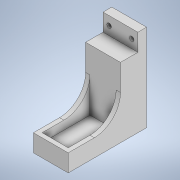
# Autodesk Inventor part: s_base8
Saved by Autodesk Inventor 2022 (Build 260153000, 153)
## iProperties
Created: 2021-09-17
Part Number: s_base8
Material: Generic
Document SubType Name: Modeling
Designer: yuto6
Density: 1 g/cm^3
Appearance: Default
Author: yuto6
Autodesk Inventor part; units mm, degrees
ref_plane "YZ Plane" through (0, 0, 0) normal (1, 0, 0) x (0, 1, 0)
ref_plane "XZ Plane" through (0, 0, 0) normal (0, 1, 0) x (-1, 0, 0)
ref_plane "XY Plane" through (0, 0, 0) normal (0, 0, 1) x (1, 0, 0)
sketch "スケッチ1" plane through (0, 0, 0) normal (1, 0, 0) x (0, 1, 0)
  line L0 (0, 0) -> (100, 0)
  line L1 (100, 0) -> (100, 10)
  line L2 (20, 90) -> (0, 90)
  line L3 (0, 90) -> (0, 0)
  line L4 (100, 10) -> (80, 10)
  line L5 (80, 10) -> (80, 30)
  line L6 (80, 30) -> (20, 30)
  line L7 (20, 30) -> (20, 90)
  dimension "d0" = 100
  dimension "d1" = 10
  dimension "d23" = 20
  dimension "d24" = 20
  dimension "d25" = 80
  dimension "d26" = 90
  constraints: 16 end point, 4 horizontal, 2 perpendicular, 2 vertical
  measures "d0" distance of L0.start L0.end
  measures "d1" distance of L0.end L1.end
  measures "d23" distance of L1.end L4.end
  measures "d24" distance of L4.end L5.end
  measures "d25" distance between parallel lines of L1 L7
  measures "d26" distance between parallel lines of L0 L2
extrude "押し出し1" add sketch "スケッチ1" along normal mid plane 40
fillet "フィレット1" radius 30 1 edges at (0, 20, 30)
sketch "スケッチ2" plane through (-20, 100, 10) normal (0, 1, 0) x (1, 0, 0)
  line L0 (0, -80) -> (40, -80) projected
  line L1 (40, -20) -> (0, -20) projected
  line L2 (5, -20) -> (35, -20)
  line L3 (35, -20) -> (35, -75)
  line L4 (35, -75) -> (5, -75)
  line L5 (5, -75) -> (5, -20)
  line L6 (0, -20) -> (0, -50) projected
  line L7 (40, -50) -> (40, -80) projected
  dimension "d27" = 5
  dimension "d28" = 5
  dimension "d29" = 5
  constraints: 8 end point, 2 parallel, 1 horizontal, 1 perpendicular, 1 point on line
  measures "d27" distance between parallel lines of L0 L4
  measures "d28" distance between parallel lines of L6 L5
  measures "d29" distance between parallel lines of L7 L3
extrude "押し出し2" cut sketch "スケッチ2" against normal blind 90
sketch "スケッチ3" plane through (20, 100, 0) normal (0, 0, -1) x (-1, 0, 0)
  line L0 (40, 0) -> (0, 0) projected
  line L1 (0, -100) -> (0, 0) projected
  line L2 (40, 0) -> (40, -100) projected
  point P0 (20, -100)
  point P1 (7, -10)
  point P2 (33, -10)
  dimension "d12" = 10
  dimension "d13" = 10
  dimension "d14" = 7
  dimension "d15" = 7
  measures "d12" distance from line of L0 point (7, -10)
  measures "d13" distance from line of L0 point (33, -10)
  measures "d14" distance from line of L1 point (7, -10)
  measures "d15" distance from line of L2 point (33, -10)
hole "穴1" at (13, 90, 0) at (-13, 90, 0) direction (0, 0, 1) diameter 5.2 end through all
equation "\"d28\" = d27"
equation "\"d29\" = d27"
equation "\"d13\" = d12"
equation "\"d15\" = d14"
